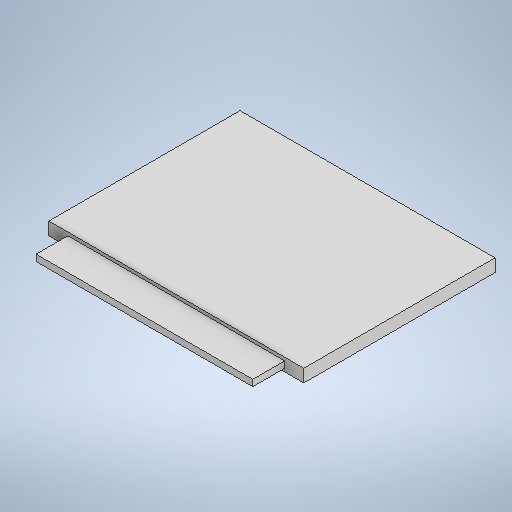
# Autodesk Inventor part: Chassis Upper
Saved by Autodesk Inventor 2025.2 (Build 292293000, 293)
## iProperties
Created: 2025-01-18
Part Number: Chassis Upper
Material: Generic
Document SubType Name: Modeling
Designer: mtidd
Density: 1 g/cm^3
Appearance: Default
Author: mtidd
Autodesk Inventor part; units mm, degrees
ref_plane "YZ Plane" through (0, 0, 0) normal (1, 0, 0) x (0, 1, 0)
ref_plane "XZ Plane" through (0, 0, 0) normal (0, 1, 0) x (-1, 0, 0)
ref_plane "XY Plane" through (0, 0, 0) normal (0, 0, 1) x (1, 0, 0)
sketch "Sketch1" plane through (0, 0, 0) normal (0, 1, 0) x (-1, 0, 0)
  line L0 (0, 0) -> (200, 0)
  line L1 (200, 0) -> (200, -300)
  line L2 (200, -300) -> (0, -300)
  line L3 (0, -300) -> (0, 0)
  line L4 (0, 0) -> (200, 0)
  line L5 (200, 0) -> (200, -150)
  line L6 (200, -150) -> (0, -150)
  line L7 (0, -150) -> (0, 0)
  dimension "d0" = 200
  dimension "d1" = 300
  dimension "d2" = 200
  dimension "d3" = 150
  constraints: 16 end point, 4 parallel, 2 horizontal, 2 perpendicular
  measures "d0" distance of L1.end L2.end
  measures "d1" distance of L0.end L1.end
  measures "d2" distance of L5.end L6.end
  measures "d3" distance of L4.end L5.end
extrude "Extrusion1" add sketch "Sketch1" along normal blind 10 contours L0 L1 L6 L3
sketch "Sketch2" plane through (-200, 0, 0) normal (0, 0, 1) x (1, 0, 0)
  line L0 (15, 2.5) -> (185, 2.5)
  line L1 (185, 2.5) -> (185, 7.5)
  line L2 (185, 7.5) -> (15, 7.5)
  line L3 (15, 7.5) -> (15, 2.5)
  point P0 (200, 0)
  dimension "d6" = 170
  dimension "d7" = 5
  constraints: 8 end point, 2 parallel, 1 horizontal, 1 perpendicular
  measures "d6" distance of L2.end L1.end
  measures "d7" distance of L1.end L0.end
extrude "Extrusion2" add sketch "Sketch2" along normal blind 25
body "Solid1"
